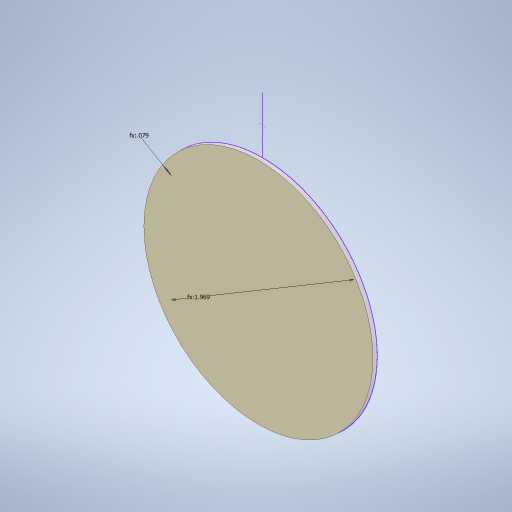
# Autodesk Inventor part: membrane
Saved by Autodesk Inventor 2023 (Build 270158000, 158)
## iProperties
Created: 2023-01-24
Part Number: membrane
Material: Generic
Document SubType Name: Modeling
Designer: remidm
Density: 1 g/cm^3
Appearance: Default
Mass: 0.506707 g
Surface Area: 10.9321 cm^2
Volume: 0.506707 cm^3
MembraneThickness: 0.039 in
Author: remidm
Autodesk Inventor part; units mm, degrees
ref_plane "YZ Plane" through (0, 0, 0) normal (1, 0, 0) x (0, 1, 0)
ref_plane "XZ Plane" through (0, 0, 0) normal (0, 1, 0) x (-1, 0, 0)
ref_plane "XY Plane" through (0, 0, 0) normal (0, 0, 1) x (1, 0, 0)
sketch "Sketch1" plane through (0, 0, 0) normal (0, 0, 1) x (1, 0, 0)
  circle A0 centre (0, 0) radius 25
  circle A1 centre (0, 0) radius 27
  line L0 (0, 33.62) -> (0, 27)
  line L1 (0, 33.62) -> (0, 40.24)
  dimension "d5" = 50
  dimension "d17" = 2
  constraints: 4 end point, 1 centre point, 1 coincident, 1 collinear, 1 point on line, 1 vertical, 1 vertical alignment, 2 other
  measures "d5" diameter of A0
extrude "Extrusion1" add sketch "Sketch1" along normal blind 1 contours A0 | A1
equation "\"d5\" = SaltDiameter"
equation "\"d17\" = crucible_thickness"
equation "\"SaltDiameter\" = 50"
equation "\"crucible_thickness\" = 2"
body "Solid1"
